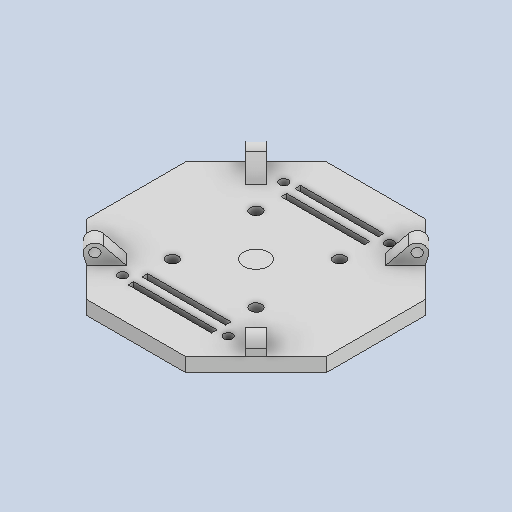
# Autodesk Inventor part: bottom
Saved by Autodesk Inventor 2025.2 (Build 292293000, 293)
## iProperties
Created: 2025-03-18
Part Number: bottom
Material: Generic
Document SubType Name: Modeling
Designer: mirewn
Density: 1 g/cm^3
Appearance: Default
Author: mirewn
Autodesk Inventor part; units mm, degrees
ref_plane "YZ Plane" through (0, 0, 0) normal (1, 0, 0) x (0, 1, 0)
ref_plane "XZ Plane" through (0, 0, 0) normal (0, 1, 0) x (-1, 0, 0)
sketch "Sketch1" plane through (0, 0, 0) normal (0, 1, 0) x (-1, 0, 0)
  line L0 (17.8112, 43) -> (43, 17.8112)
  line L1 (43, 17.8112) -> (43, -17.8112)
  line L2 (43, -17.8112) -> (17.8112, -43)
  line L3 (17.8112, -43) -> (-17.8112, -43)
  line L4 (-17.8112, -43) -> (-43, -17.8112)
  line L5 (-43, -17.8112) -> (-43, 17.8112)
  line L6 (-43, 17.8112) -> (-17.8112, 43)
  line L7 (-17.8112, 43) -> (17.8112, 43)
  point P0 (0, 0)
  point P1 (0, 0)
  point P2 (0, 43)
  dimension "d0" = 86
  constraints: 16 end point, 1 coincident, 1 midpoint, 1 vertical alignment, 17 other
  measures "d0" distance between parallel lines of L5 L1
extrude "Extrusion1" add sketch "Sketch1" along normal blind 5
sketch "Sketch3" plane through (0, 0, 0) normal (0, -1, 0) x (1, 0, 0)
  line L0 (43, 17.8112) -> (43, -17.8112) projected
  line L1 (-15, 24) -> (-15, 26)
  line L2 (-15, 26) -> (0, 26)
  line L3 (0, 29) -> (-15, 29)
  line L4 (-15, 29) -> (-15, 31)
  line L5 (-15, 31) -> (0, 31)
  line L6 (0, 0) -> (0, 24) construction
  line L7 (0, 0) -> (-3.3479, 0) construction
  line L8 (0, 24) -> (-15, 24)
  line L9 (15, 24) -> (15, 26)
  line L10 (15, 26) -> (0, 26)
  line L11 (0, 29) -> (15, 29)
  line L12 (15, 29) -> (15, 31)
  line L13 (15, 31) -> (0, 31)
  line L14 (0, 24) -> (15, 24)
  line L15 (-15, -24) -> (-15, -26)
  line L16 (-15, -26) -> (0, -26)
  line L17 (0, -29) -> (-15, -29)
  line L18 (-15, -29) -> (-15, -31)
  line L19 (-15, -31) -> (0, -31)
  line L20 (0, -24) -> (-15, -24)
  line L21 (15, -24) -> (15, -26)
  line L22 (15, -26) -> (0, -26)
  line L23 (0, -29) -> (15, -29)
  line L24 (15, -29) -> (15, -31)
  line L25 (15, -31) -> (0, -31)
  line L26 (0, -24) -> (15, -24)
  line L27 (-17.8112, 43) -> (17.8112, 43) projected
  point P0 (11.5, 17.5)
  point P1 (-15, 25)
  point P2 (-7.5, 24)
  point P3 (15, 25)
  point P4 (7.5, 24)
  point P5 (11.5, -17.5)
  point P6 (-15, -25)
  point P7 (-7.5, -24)
  point P8 (15, -25)
  point P9 (7.5, -24)
  point P10 (0, 43)
  dimension "d21" = 2
  dimension "d22" = 3
  dimension "d23" = 2
  dimension "d25" = 15
  dimension "d30" = 12
  constraints: 52 end point, 23 symmetric about line, 8 point on line, 3 midpoint, 3 perpendicular, 3 vertical alignment, 2 horizontal, 1 parallel, 1 vertical
  measures "d21" distance of L1.start L1.end
  measures "d22" distance of L2.end L3.start
  measures "d23" distance of L3.end L4.end
  measures "d25" distance from line of L1 L6.start
  measures "d30" distance from line of point (0, 43) L13
extrude "Extrusion3" cut sketch "Sketch3" against normal blind 5
sketch "Sketch4" plane through (0, 5, 0) normal (0, 1, 0) x (1, 0, 0)
  circle A0 centre (0, 0) radius 4.4721
  constraints: 1 centre point, 1 coincident
extrude "Extrusion4" cut sketch "Sketch4" against normal blind 0.01
ref_plane "Work Plane1" through (12.5944, 0, 12.5944) normal (-0.7071, 0, 0.7071) x (0.7071, 0, 0.7071)
sketch "Sketch5" plane through (12.5944, 0, 12.5944) normal (-0.7071, 0, 0.7071) x (0.7071, 0, 0.7071)
  line L0 (25.1888, 5) -> (19.1888, 5)
  line L1 (25.1888, 5) -> (0, 5)
  line L2 (19.1888, 5) -> (19.1888, 9) construction
  line L3 (19.1888, 9) -> (23.1888, 9) construction
  circle A0 centre (23.1888, 9) radius 3
  circle A1 centre (23.1888, 9) radius 1.6
  line L4 (25.1888, 5) -> (26.0788, 8.195)
  line L5 (15.1888, 5) -> (21.0249, 11.0778)
  line L6 (15.1888, 5) -> (19.1888, 5)
  line L7 (19.1888, 9.1657) -> (18.1888, 5)
  point P0 (-17.8112, 0)
  point P1 (-17.8112, 0)
  point P2 (-107.2923, -20.1826)
  point P3 (-107.2923, -23.1826)
  point P4 (15.1888, 5)
  dimension "d33" = 6
  dimension "d34" = 4
  dimension "d35" = 4
  dimension "d36" = 6
  dimension "d37" = 3.2
  dimension "d38" = 10
  dimension "d39" = 1
  constraints: 16 end point, 3 coincident, 2 centre point, 2 point on circle, 2 point on line, 2 tangent, 1 collinear, 1 perpendicular
  measures "d33" distance of L0.start L0.end
  measures "d34" distance of L0.end L2.end
  measures "d35" distance of L2.end L3.end
  measures "d36" diameter of A0
  measures "d37" diameter of A1
  measures "d38" distance of L0.start L5.start
  measures "d39" distance from line of L2 L7.end
extrude "Extrusion5" add sketch "Sketch5" along normal mid plane 5.5
pattern_circular "Circular Pattern2" count 4 over 360 about axis through (0, 5, 0) along (0, -1, 0) of "Extrusion5"
sketch "Sketch6" plane through (0, 5, 0) normal (0, 1, 0) x (1, 0, 0)
  line L0 (0, 0) -> (30.1227, 30.1227) construction
  line L1 (32.0673, 28.1782) -> (28.1782, 32.0673) construction
  line L2 (-15.05, -15.05) -> (15.05, -15.05) construction
  line L3 (15.05, -15.05) -> (15.05, 15.05) construction
  line L4 (15.05, 15.05) -> (-15.05, 15.05) construction
  line L5 (-15.05, 15.05) -> (-15.05, -15.05) construction
  line L6 (-15.05, -15.05) -> (15.05, 15.05) construction
  line L7 (15.05, -15.05) -> (-15.05, 15.05) construction
  dimension "d45" = 30.1
  dimension "d46" = 30.1
  constraints: 14 end point, 3 midpoint, 2 parallel, 1 horizontal, 1 perpendicular
  measures "d45" distance of L4.end L3.end
  measures "d46" distance of L3.end L2.end
hole "Hole1" at (-15.05, 5, -15.05) at (-15.05, 5, 15.05) at (15.05, 5, -15.05) at (15.05, 5, 15.05) direction (0, -1, 0) diameter 4.2 end through all
sketch "Sketch7" plane through (0, 5, 0) normal (0, 1, 0) x (1, 0, 0)
  line L0 (-18, -18) -> (18, -18) construction
  line L1 (18, -18) -> (18, 18) construction
  line L2 (18, 18) -> (-18, 18) construction
  line L3 (-18, 18) -> (-18, -18) construction
  line L4 (-18, -18) -> (18, 18) construction
  line L5 (18, -18) -> (-18, 18) construction
  line L6 (-19, -29) -> (19, -29) construction
  line L7 (19, -29) -> (19, 29) construction
  line L8 (19, 29) -> (-19, 29) construction
  line L9 (-19, 29) -> (-19, -29) construction
  circle A0 centre (0, 0) radius 4.4721 construction
  line L10 (-19, -29) -> (19, 29) construction
  line L11 (19, -29) -> (-19, 29) construction
  dimension "d59" = 36
  dimension "d60" = 36
  dimension "d61" = 58
  dimension "d62" = 38
  constraints: 24 end point, 4 coincident, 4 midpoint, 4 parallel, 2 horizontal, 2 perpendicular
  measures "d59" distance of L2.end L1.end
  measures "d60" distance of L1.end L0.end
  measures "d61" distance of L8.end L6.start
  measures "d62" distance of L7.end L8.end
hole "Hole2" at (-19, 5, -29) at (19, 5, -29) at (19, 5, 29) at (-19, 5, 29) direction (0, -1, 0) diameter 3.2 end through all
body "Solid1"
